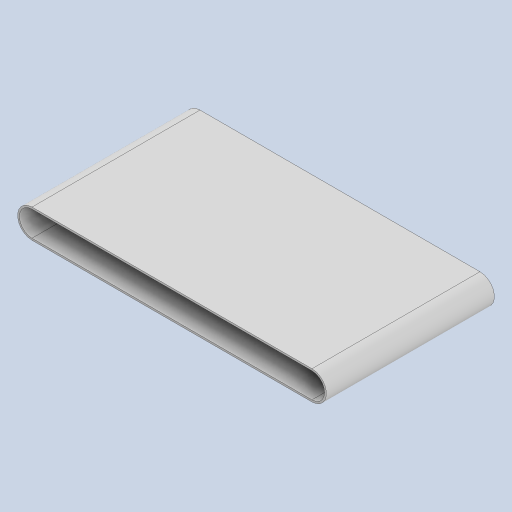
# Autodesk Inventor part: belt
Saved by Autodesk Inventor 2024 (Build 280153000, 153)
## iProperties
Created: 2023-05-24
Part Number: belt
Material: Generic
Document SubType Name: Modeling
Designer: pc
Density: 1 g/cm^3
Appearance: Default
Author: pc
Autodesk Inventor part; units mm, degrees
ref_plane "YZ Plane" through (0, 0, 0) normal (1, 0, 0) x (0, 1, 0)
ref_plane "XZ Plane" through (0, 0, 0) normal (0, 1, 0) x (-1, 0, 0)
ref_plane "XY Plane" through (0, 0, 0) normal (0, 0, 1) x (1, 0, 0)
sketch "Sketch1" plane through (0, 0, 0) normal (0, 0, 1) x (1, 0, 0)
  line L0 (-395.8181, -42.4329) -> (366.1819, -42.4329) projected
  line L1 (-395.8181, -102.4277) -> (366.1819, -102.4277) projected
  arc A0 (366.1819, -102.4277) -> (366.1819, -42.4329) centre (366.1819, -72.4303) ccw
  arc A1 (-395.8181, -42.4329) -> (-395.8181, -102.4277) centre (-395.8181, -72.4303) ccw
  line L2 (366.1819, -38.2063) -> (-395.8181, -38.2063)
  arc A2 (-395.8181, -38.2063) -> (-395.8181, -106.6542) centre (-395.8181, -72.4303) ccw
  line L3 (-395.8181, -106.6542) -> (366.1819, -106.6542)
  arc A3 (366.1819, -106.6542) -> (366.1819, -38.2063) centre (366.1819, -72.4303) ccw
  line L4 (-395.8181, -33.2473) -> (366.1819, -33.2473)
  arc A4 (366.1819, -111.6132) -> (366.1819, -33.2473) centre (366.1819, -72.4303) ccw
  line L5 (366.1819, -111.6132) -> (-395.8181, -111.6132)
  arc A5 (-395.8181, -33.2473) -> (-395.8181, -111.6132) centre (-395.8181, -72.4303) ccw
  point P0 (0, 0)
  point P1 (-397.2939, -72.395)
  constraints: 12 end point, 12 point on circle, 6 centre point, 3 tangent, 1 coincident, 6 other
extrude "Extrusion1" add sketch "Sketch1" along normal blind 203.2 and the other way blind 254 contours L4 A4 L5 A5
sketch "Sketch2" plane through (-395.8181, -106.6542, 203.2) normal (0, 1, 0) x (1, 0, 0)
  point P0 (395.8181, 203.2)
sketch "Sketch3" plane through (-395.8181, -33.2473, 203.2) normal (0, 1, 0) x (1, 0, 0)
  line L0 (0, 457.2) -> (762, 457.2) projected
  line L1 (381, 457.2) -> (381, 355.6)
  line L2 (381, 0.2737) -> (381, 101.8737)
  line L3 (0, 457.2) -> (0, 0) projected
  line L4 (0, 355.6) -> (762, 355.6)
  line L5 (762, 355.6) -> (762, 101.8737)
  line L6 (762, 101.8737) -> (0, 101.8737)
  line L7 (0, 101.8737) -> (0, 355.6)
  point P0 (395.8181, 203.2)
  dimension "d4" = 101.6
  dimension "d5" = 101.6
  constraints: 12 end point, 2 parallel, 2 perpendicular, 2 vertical, 1 midpoint, 1 point on line
  measures "d4" distance of L1.start L1.end
  measures "d5" distance of L2.start L2.end
extrude "Extrusion2" [suppressed]
body "Solid1"
